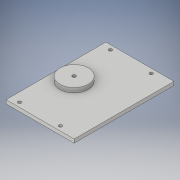
# Autodesk Inventor part: Slider
Saved by Autodesk Inventor 2019 (Build 230136000, 136)
## iProperties
Created: 2020-04-04
Part Number: Slider
Material: Generic
Document SubType Name: Modeling
Designer: james
Density: 1 g/cm^3
Appearance: Default
Author: james
Autodesk Inventor part; units mm, degrees
ref_plane "YZ Plane" through (0, 0, 0) normal (1, 0, 0) x (0, 1, 0)
ref_plane "XZ Plane" through (0, 0, 0) normal (0, 1, 0) x (-1, 0, 0)
ref_plane "XY Plane" through (0, 0, 0) normal (0, 0, 1) x (1, 0, 0)
sketch "Sketch1" plane through (0, 0, 0) normal (0, 1, 0) x (-1, 0, 0)
  line L0 (56.2338, 50.9905) -> (-39.0162, 50.9905)
  line L1 (-39.0162, 50.9905) -> (-39.0162, -88.7095)
  line L2 (-39.0162, -88.7095) -> (56.2338, -88.7095)
  line L3 (56.2338, -88.7095) -> (56.2338, 50.9905)
  point P0 (0, 0)
  dimension "d0" = 139.7
  dimension "d1" = 95.25
  constraints: 8 end point, 2 parallel, 1 horizontal, 1 perpendicular
  measures "d0" distance of L0.end L1.end
  measures "d1" distance of L0.start L0.end
extrude "Extrusion1" add sketch "Sketch1" along normal blind 5.08
sketch "Sketch2" plane through (0, 5.08, 0) normal (0, 1, 0) x (1, 0, 0)
  line L0 (-56.2338, -50.9905) -> (39.0162, -50.9905) projected
  line L1 (39.0162, 88.7095) -> (-56.2338, 88.7095) projected
  line L2 (-56.2338, 88.7095) -> (-56.2338, -50.9905) projected
  point P0 (0, 0)
  point P1 (-43.5338, -44.6405)
  point P2 (13.6162, -44.6405)
  point P3 (13.6162, 82.3595)
  point P4 (-43.5338, 82.3595)
  dimension "d4" = 0
  dimension "d5" = 6.35
  dimension "d6" = 0
  dimension "d7" = 6.35
  dimension "d8" = 0
  dimension "d9" = 0
  dimension "d10" = 12.7
  dimension "d11" = 57.15
  measures "d4" vertical distance of point (13.616, -44.641) point (-43.534, -44.641)
  measures "d5" distance from line of L0 point (13.616, -44.641)
  measures "d6" vertical distance of point (-43.534, 82.359) point (13.616, 82.359)
  measures "d7" distance from line of L1 point (-43.534, 82.359)
  measures "d8" horizontal distance of point (-43.534, 82.359) point (-43.534, -44.641)
  measures "d9" horizontal distance of point (13.616, -44.641) point (13.616, 82.359)
  measures "d10" distance from line of L2 point (-43.534, -44.641)
  measures "d11" distance of point (13.616, -44.641) point (-43.534, -44.641)
hole "Hole1" at (-43.5338, 5.08, 44.6405) at (13.6162, 5.08, 44.6405) at (13.6162, 5.08, -82.3595) at (-43.5338, 5.08, -82.3595) direction (0, -1, 0) diameter 4.4958 end through all clearance for "Flat Head Machine Screw (82)" size "#8" standard "Ansi Unified Screw Threads"
sketch "Sketch4" plane through (0, 5.08, 0) normal (0, 1, 0) x (1, 0, 0)
  circle A0 centre (-30.8338, 18.8595) radius 19.8293
  line L0 (-56.2338, -50.9905) -> (39.0162, -50.9905) projected
  line L1 (-56.2338, 88.7095) -> (-56.2338, -50.9905) projected
  point P0 (0, 0)
  dimension "d26" = 69.85
  dimension "d27" = 25.4
  constraints: 1 centre point
  measures "d26" distance from line of L0 A0.centre
  measures "d27" distance from line of L1 A0.centre
extrude "Extrusion3" add sketch "Sketch4" along normal blind 6.35
sketch "Sketch5" plane through (-30.8338, 11.43, -18.8595) normal (0, 1, 0) x (1, 0, 0)
  circle A0 centre (0, 0) radius 2.3813
  point P0 (30.8338, -18.8595)
  dimension "d30" = 4.7625
  constraints: 1 centre point
  measures "d30" diameter of A0
extrude "Extrusion4" cut sketch "Sketch5" against normal blind 33.3375
sketch "Sketch6" plane through (0, 0, 0) normal (0, -1, 0) x (1, 0, 0)
  circle A0 centre (-30.8338, -18.8595) radius 2.3813 projected
  circle A1 centre (-30.8338, -18.8595) radius 9.525
  point P0 (0, 0)
  dimension "d33" = 19.05
  constraints: 1 centre point, 1 coincident
  measures "d33" diameter of A1
extrude "Extrusion5" cut sketch "Sketch6" against normal blind 5.08
body "Solid1"
